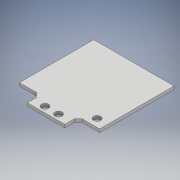
# Autodesk Inventor part: pixy
Saved by Autodesk Inventor 2017 (Build 210142000, 142)
## iProperties
Part Number: pixy
Material: 一般
Document SubType Name: Modeling
Designer: highs
Density: 1 g/cm^3
Appearance: 既定
Author: highs
Autodesk Inventor part; units mm, degrees
ref_plane "YZ Plane" through (0, 0, 0) normal (1, 0, 0) x (0, 1, 0)
ref_plane "XZ Plane" through (0, 0, 0) normal (0, 1, 0) x (-1, 0, 0)
ref_plane "XY Plane" through (0, 0, 0) normal (0, 0, 1) x (1, 0, 0)
sketch "スケッチ1" plane through (0, 0, 0) normal (0, 0, 1) x (1, 0, 0)
  line L0 (0, 0) -> (17.8, 0)
  line L1 (17.8, 0) -> (17.8, 6.4)
  line L2 (17.8, 6.4) -> (28, 6.4)
  line L3 (28, 6.4) -> (28, 41.8)
  line L4 (28, 41.8) -> (-10.2, 41.8)
  line L5 (-10.2, 41.8) -> (-10.2, 6.4)
  line L6 (-10.2, 6.4) -> (0, 6.4)
  line L7 (0, 6.4) -> (0, 0)
  line L8 (0, 2.7) -> (17.8, 2.7) construction
  circle A0 centre (5.7, 2.7) radius 1.7
  circle A1 centre (12.1, 2.7) radius 1.7
  circle A2 centre (23.1, 10.1) radius 1.7
  dimension "d0" = 3.4
  dimension "d1" = 17.8
  dimension "d2" = 6.4
  dimension "d3" = 5.7
  dimension "d4" = 2.7
  dimension "d5" = 6.4
  dimension "d6" = 35.4
  dimension "d7" = 38.2
  dimension "d8" = 10.2
  dimension "d9" = 4.9
  dimension "d10" = 3.7
  constraints: 18 end point, 7 perpendicular, 6 point on line, 3 centre point, 2 equal radius, 1 horizontal
  measures "d0" diameter of A0
  measures "d1" distance of L0.start L0.end
  measures "d2" distance of A1.centre A0.centre
  measures "d3" distance from line of L7 A0.centre
  measures "d4" distance between parallel lines of L0 L8
  measures "d5" distance of L6.end L0.start
  measures "d6" distance of L4.end L5.end
  measures "d7" distance of L3.end L4.end
  measures "d8" distance of L5.end L6.end
  measures "d9" distance from line of L3 A2.centre
  measures "d10" distance from line of L2 A2.centre
extrude "押し出し1" add sketch "スケッチ1" along normal blind 1.5
chamfer "面取り1" distance 2 angle 45 2 edges at (17.8, 6.4, 0.75) (0, 6.4, 0.75)
